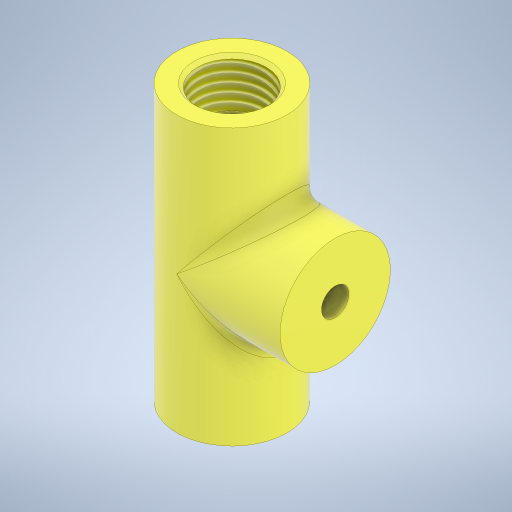
# Autodesk Inventor part: 1 HUDSON-8-28B-TDR HAND PUMP BASE BODY
Saved by Autodesk Inventor 2024.2 (Build 282272000, 272)
## iProperties
Created: 2024-11-13
Part Number: 1 HUDSON-8-28B-TDR HAND PUMP BASE BODY
Material: Genérico
Document SubType Name: Modeling
Designer: brene
Density: 1 g/cm^3
Appearance: Suave - Amarillo
Author: brene
Autodesk Inventor part; units mm, degrees
ref_plane "YZ Plane" through (0, 0, 0) normal (1, 0, 0) x (0, 1, 0)
ref_plane "XZ Plane" through (0, 0, 0) normal (0, 1, 0) x (-1, 0, 0)
sketch "Boceto1" plane through (0, 0, 0) normal (0, 0, 1) x (1, 0, 0)
  line L0 (-53.3198, 0) -> (53.3198, 0)
  line L1 (0, 30.5381) -> (0, -30.5381)
  line L2 (0, 20) -> (8, 20)
  line L3 (8, 20) -> (8, 9.2995)
  line L4 (8, 9.2995) -> (8, 8)
  line L5 (8, 8) -> (15, 8)
  line L6 (8, -20) -> (0, -20)
  line L7 (5, 20) -> (5, 13)
  line L8 (5, 13) -> (4, 13)
  line L9 (4, 13) -> (4, 8)
  line L10 (4, 8) -> (4, 6)
  line L11 (4, 6) -> (15, 6)
  line L12 (4, -6) -> (4, -12)
  line L13 (15, -8) -> (8, -8)
  line L14 (15, 8) -> (15, 6)
  line L15 (4, 6) -> (2, 6)
  line L16 (2, 6) -> (2, 0.2831)
  line L17 (2, 0.2831) -> (2, -4.2831)
  line L18 (5, -20) -> (5, -12)
  line L19 (5, -12) -> (4, -12)
  line L20 (2, -4.2831) -> (2, -5.0525)
  line L21 (4, -6) -> (2, -5.0525)
  line L22 (8, -20) -> (8, -8)
  line L23 (15, -8) -> (15, 6)
  line L24 (2, -2) -> (15, -2)
  line L25 (15, 2) -> (2, 2)
  line L26 (8, 8) -> (8, -8)
  point P0 (0, 0)
  point P1 (0, 0)
  point P2 (15, 0)
  point P3 (8, -2)
  point P4 (8, 2)
  dimension "d0" = 16
  dimension "d4" = 7
  dimension "d7" = 7
  dimension "d8" = 10
  dimension "d9" = 8
  dimension "d10" = 7
  dimension "d12" = 2
  dimension "d13" = 4
  dimension "d15" = 20
  dimension "d16" = 20
  dimension "d17" = 14
  dimension "d18" = 8
  dimension "d19" = 10
  dimension "d20" = 8
  dimension "d21" = 7
  dimension "d22" = 4
  dimension "d23" = 16
  dimension "d24" = 4
  dimension "d25" = 25.348
  dimension "d26" = 8
  dimension "d27" = 38.3198
  dimension "d28" = 0
  dimension "d29" = 1.2995
  dimension "d30" = 7.7169
  dimension "d31" = 22.5381
  constraints: 54 end point, 13 point on line, 10 perpendicular, 6 vertical, 3 horizontal, 3 midpoint, 2 parallel, 1 coincident
  measures "d0" diameter of L3 L1
  measures "d4" distance of L4.end L5.end
  measures "d7" distance of L7.start L7.end
  measures "d8" diameter of L7 L1
  measures "d9" diameter of L9 L1
  measures "d10" distance of L8.end L10.end
  measures "d12" distance of L10.end L15.end
  measures "d13" diameter of L16 L1
  measures "d15" vertical distance of point (15, 0) L2.end
  measures "d16" vertical distance of L6.start point (15, 0)
  measures "d17" vertical distance of L6.start L12.start
  measures "d18" diameter of L12 L1
  measures "d19" diameter of L18 L1
  measures "d20" distance of L18.start L18.end
  measures "d21" distance of L13.start L13.end
  measures "d22" diameter of L24 L0
  measures "d23" diameter of L5 L0
  measures "d24" diameter of L25 L0
  measures "d25" angle of L21 L5
  measures "d26" distance from line of point (0, 0) L13
  measures "d27" distance from line of L0.end L23
  measures "d28" distance from line of point (15, 0) L23
  measures "d29" distance from line of L3.end L5
  measures "d30" distance from line of L16.end L5
  measures "d31" distance from line of L1.start L5
revolve "Revolución1" add sketch "Boceto1" angle 360 about axis through (0, 30.5381, 0) along (0, -1, 0) contours L17 L16 L25 L26 L0 | L0 L26 L24 L17 | L24 L26 L22 L6 L18 L19 L12 L21 L20 L17 | L2 L3 L4 L26 L11 L10 L9 L8 L7 | L25 L16 L15 L11 L26
revolve "Revolución2" add sketch "Boceto1" angle 360 about axis through (-53.3198, 0, 0) along (1, 0, 0) contours L26 L11 L23 L25 | L24 L23 L13 L26 | L26 L5 L14 L11
sketch "Boceto2" plane through (8, 0, 0) normal (-1, 0, 0) x (0, 0, 1)
  circle A0 centre (0, 0) radius 8
  point P0 (0, 0)
  dimension "d36" = 16
  constraints: 1 centre point, 1 coincident
  measures "d36" diameter of A0
extrude "Extrusión1" add sketch "Boceto2" along normal blind 4
sketch "Boceto3" plane through (8, 0, 0) normal (1, 0, 0) x (0, 0, -1)
  circle A0 centre (0, 0) radius 2
  dimension "d37" = 4
  constraints: 1 centre point, 1 coincident
  measures "d37" diameter of A0
extrude "Extrusión2" cut sketch "Boceto3" against normal blind 8
thread "Rosca1" size "M10x1.25" class "6H" standard "ANSI Metric M Profile" length 7
chamfer "Chaflán1" distance 0.5 angle 45 2 edges at (-5, 20, 0) (-5, -20, 0)
sketch "Boceto4" plane through (4, 0, 0) normal (-1, 0, 0) x (0, 0, 1)
  line L0 (-5.3914, -4.0896) -> (-5.3914, 5.9104)
  line L1 (4.9189, 6.3091) -> (4.9189, -3.6909)
  circle A0 centre (0, 0) radius 8
  line L2 (-5.3914, -4.0896) -> (-5.3914, -5.9104)
  line L3 (4.9189, -3.6909) -> (4.9189, -6.3091)
  point P0 (-5.3914, 5.9104)
  dimension "d49" = 10
  dimension "d50" = 10
  dimension "d68" = 16
  dimension "d69" = 10.3103
  dimension "d70" = 4.9189
  dimension "d71" = 12.6182
  dimension "d72" = 10.318
  constraints: 8 end point, 2 parallel, 2 point on circle, 2 vertical, 1 centre point
  measures "d49" distance of L1.start L1.end
  measures "d50" distance of L0.start L0.end
  measures "d68" diameter of A0
  measures "d69" distance between parallel lines of L1 L0
  measures "d70" distance from line of A0.centre L1
  measures "d71" distance of L1.start L3.end
  measures "d72" distance of L1.start L0.end
extrude "Extrusión4" add sketch "Boceto4" along normal blind 4 contours L2 A0 L0 | A0 L3 L1
ref_plane "Plano de trabajo1" through (-53.3198, 0, 0) normal (0, 0, -1) x (1, 0, 0)
thread "Rosca2" size "M10x1.25" class "6H" standard "ANSI Metric M Profile" length 7
fillet "Empalme2" radius 2 8 edges at (6.9282, 6.9282, 4) (2.0706, 2.0706, 7.7274) (2.0706, 2.0706, -7.7274) (6.9282, 6.9282, -4) (2.0706, -2.0706, 7.7274) (6.9282, -6.9282, 4) (6.9282, -6.9282, -4) (2.0706, -2.0706, -7.7274)
equation "\"d50\" = d49"
